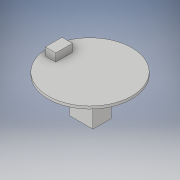
# Autodesk Inventor part: circular disc and servos
Saved by Autodesk Inventor 2019 (Build 230136000, 136)
## iProperties
Created: 2020-04-13
Part Number: circular disc and servos
Material: Generic
Document SubType Name: Modeling
Designer: DISHA PATIL
Density: 1 g/cm^3
Appearance: Default
Author: DISHA PATIL
Autodesk Inventor part; units mm, degrees
ref_plane "YZ Plane" through (0, 0, 0) normal (1, 0, 0) x (0, 1, 0)
ref_plane "XZ Plane" through (0, 0, 0) normal (0, 1, 0) x (-1, 0, 0)
ref_plane "XY Plane" through (0, 0, 0) normal (0, 0, 1) x (1, 0, 0)
sketch "Sketch1" plane through (0, 0, 0) normal (0, 1, 0) x (-1, 0, 0)
  circle A0 centre (0, 0) radius 80
  dimension "d0" = 160
  constraints: 1 centre point, 1 coincident
  measures "d0" diameter of A0
extrude "Extrusion1" add sketch "Sketch1" along normal blind 5
sketch "Sketch2" plane through (0, 5, 0) normal (0, 1, 0) x (1, 0, 0)
  line L0 (-69.1444, -16.468) -> (-49.1444, -16.468)
  line L1 (-49.1444, -16.468) -> (-49.1444, 15.532)
  line L2 (-49.1444, 15.532) -> (-69.1444, 15.532)
  line L3 (-69.1444, 15.532) -> (-69.1444, -16.468)
  point P0 (0, 0)
  dimension "d3" = 20
  dimension "d4" = 32
  constraints: 8 end point, 2 parallel, 1 horizontal, 1 perpendicular
  measures "d3" distance of L2.end L1.end
  measures "d4" distance of L1.end L0.end
extrude "Extrusion2" add sketch "Sketch2" along normal blind 15
sketch "Sketch3" plane through (0, 0, 0) normal (0, -1, 0) x (1, 0, 0)
  line L0 (22.6962, 17.1014) -> (-22.3038, 17.1014)
  line L1 (-22.3038, 17.1014) -> (-22.3038, -17.8986)
  line L2 (-22.3038, -17.8986) -> (22.6962, -17.8986)
  line L3 (22.6962, -17.8986) -> (22.6962, 17.1014)
  point P0 (0, 0)
  dimension "d7" = 45
  dimension "d8" = 35
  constraints: 8 end point, 2 parallel, 1 horizontal, 1 perpendicular
  measures "d7" distance of L2.end L1.end
  measures "d8" distance of L1.end L0.end
extrude "Extrusion3" add sketch "Sketch3" along normal blind 70
sketch "Sketch4" plane through (-49.1444, 5, -15.532) normal (0, 0, -1) x (-1, 0, 0)
  point P0 (-49.1444, -5)
body "Solid1"
